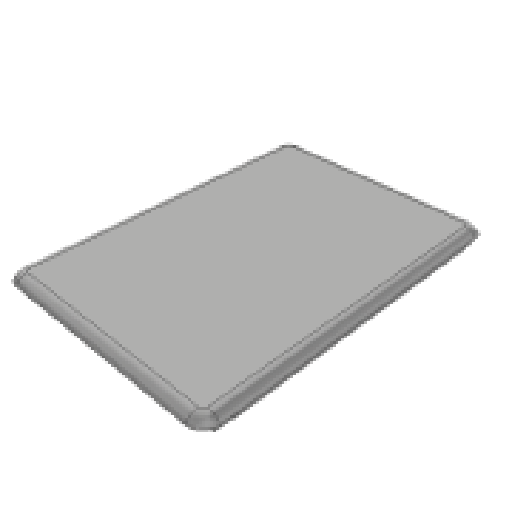
# Autodesk Inventor part: dellLatitudeScreen
Saved by Autodesk Inventor 2025 (Build 290162000, 162)
## iProperties
Created: 2024-12-07
Part Number: dellLatitudeScreen
Material: Generic
Document SubType Name: Modeling
Designer: derm
Density: 1 g/cm^3
Appearance: Smooth - Medium Gray
Author: derm
Autodesk Inventor part; units mm, degrees
ref_plane "YZ Plane" through (0, 0, 0) normal (1, 0, 0) x (0, 1, 0)
ref_plane "XZ Plane" through (0, 0, 0) normal (0, 1, 0) x (-1, 0, 0)
ref_plane "XY Plane" through (0, 0, 0) normal (0, 0, 1) x (1, 0, 0)
sketch "Sketch1" plane through (0, 0, 0) normal (0, 1, 0) x (-1, 0, 0)
  line L0 (-101.6, 165.1) -> (101.6, 165.1)
  line L1 (117.475, 149.225) -> (117.475, -149.225)
  line L2 (101.6, -165.1) -> (-101.6, -165.1)
  line L3 (-117.475, -149.225) -> (-117.475, 149.225)
  line L4 (-117.475, 165.1) -> (117.475, -165.1) construction
  line L5 (117.475, 165.1) -> (-117.475, -165.1) construction
  arc A0 (-101.6, 165.1) -> (-117.475, 149.225) centre (-101.6, 149.225) ccw
  arc A1 (-117.475, -149.225) -> (-101.6, -165.1) centre (-101.6, -149.225) ccw
  arc A2 (101.6, -165.1) -> (117.475, -149.225) centre (101.6, -149.225) ccw
  arc A3 (117.475, 149.225) -> (101.6, 165.1) centre (101.6, 149.225) ccw
  point P0 (0, 0)
  point P1 (0, 0)
  dimension "d0" = 330.2
  dimension "d1" = 234.95
  dimension "d2" = 15.875
  constraints: 12 end point, 8 point on circle, 8 point on line, 8 tangent, 4 centre point, 3 equal radius, 2 midpoint, 2 parallel, 1 coincident, 1 horizontal, 1 perpendicular
  measures "d0" distance of L5.start L4.end
  measures "d1" distance between parallel lines of L3 L1
  measures "d2" radius of A0
extrude "Extrusion1" add sketch "Sketch1" along normal blind 7.6835
fillet "Fillet1" radius 12.7 8 edges at (117.475, 7.6835, 0) (112.8253, 7.6835, -160.4503) (0, 7.6835, -165.1) (-112.8253, 7.6835, -160.4503) (-117.475, 7.6835, 0) (-112.8253, 7.6835, 160.4503) (0, 7.6835, 165.1) (112.8253, 7.6835, 160.4503)
sketch "Sketch2" plane through (0, 0, 0) normal (0, -1, 0) x (1, 0, 0)
  line L0 (101.6103, 150.8125) -> (101.6103, -150.8125) projected
  arc A0 (101.6103, 150.8125) -> (101.6, 150.8228) centre (101.6, 150.8125) ccw projected
  line L1 (-101.6, 150.8228) -> (101.6, 150.8228) projected
  arc A1 (-101.6, 150.8228) -> (-101.6103, 150.8125) centre (-101.6, 150.8125) ccw projected
  line L2 (-101.6103, -150.8125) -> (-101.6103, 150.8125) projected
  arc A2 (-101.6103, -150.8125) -> (-101.6, -150.8228) centre (-101.6, -150.8125) ccw projected
  line L3 (101.6, -150.8228) -> (-101.6, -150.8228) projected
  arc A3 (101.6, -150.8228) -> (101.6103, -150.8125) centre (101.6, -150.8125) ccw projected
  line L4 (103.505, -134.9375) -> (117.475, -134.9375) projected
  line L5 (117.475, -134.9375) -> (117.475, -150.8125) projected
  arc A4 (101.6, -166.6875) -> (117.475, -150.8125) centre (101.6, -150.8125) ccw projected
  line L6 (101.6, -166.6875) -> (-101.6, -166.6875) projected
  arc A5 (-117.475, -150.8125) -> (-101.6, -166.6875) centre (-101.6, -150.8125) ccw projected
  line L7 (-117.475, -150.8125) -> (-117.475, 150.8125) projected
  arc A6 (-101.6, 166.6875) -> (-117.475, 150.8125) centre (-101.6, 150.8125) ccw projected
  line L8 (-101.6, 166.6875) -> (101.6, 166.6875) projected
  arc A7 (117.475, 150.8125) -> (101.6, 166.6875) centre (101.6, 150.8125) ccw projected
  line L9 (117.475, 150.8125) -> (117.475, 134.9375) projected
  line L10 (117.475, 134.9375) -> (103.505, 134.9375) projected
  line L11 (103.505, 134.9375) -> (103.505, -134.9375) projected
  circle A8 centre (76.6206, 156.377) radius 5.1319 projected
  line L12 (-38.4175, -52.3875) -> (-38.4175, 52.3875) projected
  line L13 (-38.4175, 52.3875) -> (-104.4575, 52.3875) projected
  line L14 (-104.4575, 52.3875) -> (-104.4575, -52.3875) projected
  line L15 (-104.4575, -52.3875) -> (-38.4175, -52.3875) projected
  line L16 (88.265, -146.05) -> (88.265, 146.05) projected
  line L17 (88.265, 146.05) -> (-28.8925, 146.05) projected
  line L18 (-28.8925, 146.05) -> (-28.8925, -146.05) projected
  line L19 (-28.8925, -146.05) -> (88.265, -146.05) projected
  line L20 (104.922, 134.9375) -> (117.475, 134.9375)
  line L21 (117.475, 134.9375) -> (117.475, -134.9375)
  line L22 (117.475, -134.9375) -> (104.922, -134.9375)
  line L23 (104.922, -134.9375) -> (104.922, 134.9375)
  point P0 (0, 0)
  constraints: 8 end point, 2 parallel, 1 horizontal, 1 perpendicular, 1 point on line
extrude "Extrusion2" add sketch "Sketch2" along normal blind 12.7 contours L23 L10 L21 L4
sketch "Sketch4" plane through (0, 0, 0) normal (0, 0, 1) x (1, 0, 0)
  circle A0 centre (109.8636, -6.6929) radius 3.8393 projected
  circle A1 centre (109.8636, -6.6929) radius 3.8393 projected
  point P0 (0, 0)
extrude "Extrusion3" add sketch "Sketch4" along normal mid plane 300
fillet "Fillet2" radius 12.7 1 edges at (117.475, -12.7, 0)
fillet "Fillet3" radius 3.175 1 edges at (104.922, -12.6991, 0)
sketch "Sketch5" plane through (0, 0, 0) normal (0, -1, 0) x (1, 0, 0)
  line L0 (104.922, 134.9375) -> (117.475, 134.9375) projected
  line L1 (117.475, 149.225) -> (117.475, 134.9375) projected
  arc A0 (117.475, 149.225) -> (101.6, 165.1) centre (101.6, 149.225) ccw projected
  line L2 (-101.6, 165.1) -> (101.6, 165.1) projected
  arc A1 (-101.6, 165.1) -> (-117.475, 149.225) centre (-101.6, 149.225) ccw projected
  line L3 (-117.475, -149.225) -> (-117.475, 149.225) projected
  arc A2 (-117.475, -149.225) -> (-101.6, -165.1) centre (-101.6, -149.225) ccw projected
  line L4 (101.6, -165.1) -> (-101.6, -165.1) projected
  arc A3 (101.6, -165.1) -> (117.475, -149.225) centre (101.6, -149.225) ccw projected
  line L5 (117.475, -134.9375) -> (117.475, -149.225) projected
  line L6 (117.475, -134.9375) -> (104.922, -134.9375) projected
  line L7 (104.922, -134.9375) -> (104.922, 134.9375) projected
  line L8 (89.535, -147.32) -> (-92.075, -147.32)
  line L9 (-92.075, -147.32) -> (-92.075, 147.32)
  line L10 (-92.075, 147.32) -> (89.535, 147.32)
  line L11 (89.535, 147.32) -> (89.535, -147.32)
  line L12 (89.535, -147.32) -> (-92.075, 147.32) construction
  line L13 (-92.075, -147.32) -> (89.535, 147.32) construction
  circle A4 centre (-103.4539, 0) radius 1.8839
  point P0 (0, 0)
  point P1 (-1.27, 0)
  dimension "d12" = 17.78
  dimension "d13" = 17.78
  dimension "d14" = 25.4
  dimension "d15" = 27.94
  constraints: 12 end point, 2 midpoint, 2 parallel, 1 centre point, 1 horizontal, 1 perpendicular
  measures "d12" distance between parallel lines of L2 L10
  measures "d13" distance between parallel lines of L4 L8
  measures "d14" distance between parallel lines of L3 L9
  measures "d15" distance between parallel lines of L11 L5
extrude "Extrusion4" cut sketch "Sketch5" against normal blind 0.254 contours L8 L9 L10 L11 | A4
body "Solid1"
